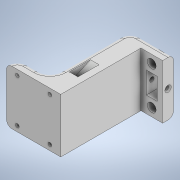
# Autodesk Inventor part: Joint_Tubes_1_2
Saved by Autodesk Inventor 2022.3 (Build 263350000, 350)
## iProperties
Created: 2023-03-29
Part Number: Joint_Tubes_1_2
Material: Generic
Document SubType Name: Modeling
Designer: Manuel Hueso Béjar
Density: 1 g/cm^3
Appearance: Default
Author: Manuel Hueso Béjar
Autodesk Inventor part; units mm, degrees
ref_plane "YZ Plane" through (0, 0, 0) normal (1, 0, 0) x (0, 1, 0)
ref_plane "XZ Plane" through (0, 0, 0) normal (0, 1, 0) x (-1, 0, 0)
ref_plane "XY Plane" through (0, 0, 0) normal (0, 0, 1) x (1, 0, 0)
sketch "Sketch1" plane through (0, 0, 0) normal (0, 1, 0) x (-1, 0, 0)
  line L0 (-10, 37) -> (10, 37)
  line L1 (10, 37) -> (10, -37)
  line L2 (10, -37) -> (-10, -37)
  line L3 (-10, -37) -> (-10, 37)
  line L4 (-10, 37) -> (10, -37) construction
  line L5 (10, 37) -> (-10, -37) construction
  line L6 (-10, 37) -> (40, 37)
  line L7 (40, 37) -> (40, 27)
  line L8 (40, 27) -> (-10, 27)
  line L9 (-10, 27) -> (-10, 37)
  line L10 (10, -37) -> (-30, -37)
  line L11 (-30, -37) -> (-30, -47)
  line L12 (-30, -47) -> (10, -47)
  line L13 (10, -47) -> (10, -37)
  point P0 (0, 0)
  point P1 (-10, -37)
  point P2 (10, 27)
  dimension "d0" = 20
  dimension "d1" = 74
  dimension "d2" = 50
  dimension "d3" = 10
  dimension "d4" = 40
  dimension "d5" = 10
  constraints: 28 end point, 6 parallel, 3 horizontal, 3 perpendicular, 2 midpoint
  measures "d0" distance of L1.end L2.end
  measures "d1" distance of L0.end L1.end
  measures "d2" distance of L7.end L8.end
  measures "d3" distance of L6.end L7.end
  measures "d4" distance of L12.end L11.end
  measures "d5" distance of L11.end L10.end
extrude "Extrusion1" add sketch "Sketch1" along normal blind 50
fillet "Fillet1" radius 10 2 edges at (-10, 25, -47) (-10, 25, 27)
fillet "Fillet2" radius 5 12 edges at (15, 50, -47) (-10, 50, -9.9999) (-12.9289, 50, 24.0711) (-29.9999, 50, 27) (-7.0711, 50, -44.0711) (-7.0711, 0, -44.0711) (-10, 0, -9.9999) (-12.9289, 0, 24.0711) (-29.9999, 0, 27) (15, 0, -47) (-40, 50, 32) (-40, 0, 32)
fillet "Fillet3" radius 10 3 edges at (-38.5355, 48.5355, 28.4645) (-38.5355, 1.4645, 28.4645) (-40, 25, 27)
sketch "Sketch2" plane through (10, 0, 37) normal (0, 0, 1) x (1, 0, 0)
  line L0 (0, 50) -> (-10, 50)
  line L1 (-10, 50) -> (-10, 45)
  line L2 (-10, 45) -> (0, 45)
  line L3 (0, 45) -> (0, 50)
  line L4 (-10, 0) -> (-10, 5) projected
  line L5 (0, 0) -> (-10, 0)
  line L6 (-10, 0) -> (-10, 5)
  line L7 (-10, 5) -> (0, 5)
  line L8 (0, 5) -> (0, 0)
  line L9 (0, 50) -> (-40, 50)
  line L10 (-40, 50) -> (-40, 45)
  line L11 (-40, 45) -> (0, 45)
  line L12 (0, 45) -> (0, 50)
  line L13 (0, 0) -> (-40, 0)
  line L14 (-40, 0) -> (-40, 5)
  line L15 (-40, 5) -> (0, 5)
  line L16 (0, 5) -> (0, 0)
  circle A0 centre (-10, 5) radius 1.7
  circle A1 centre (-10, 45) radius 1.7
  circle A2 centre (-40, 5) radius 1.7
  circle A3 centre (-40, 45) radius 1.7
  dimension "d11" = 10
  dimension "d12" = 5
  dimension "d13" = 10
  dimension "d14" = 5
  dimension "d15" = 40
  dimension "d16" = 5
  dimension "d17" = 40
  dimension "d18" = 5
  dimension "d19" = 3.4
  dimension "d20" = 3.4
  dimension "d21" = 3.4
  dimension "d22" = 3.4
  constraints: 32 end point, 8 parallel, 4 centre point, 4 coincident, 4 horizontal, 4 perpendicular
  measures "d11" distance of L2.end L1.end
  measures "d12" distance of L1.end L0.end
  measures "d13" distance of L4.end L7.end
  measures "d14" distance of L5.end L4.end
  measures "d15" distance of L11.end L10.end
  measures "d16" distance of L10.end L9.end
  measures "d17" distance of L14.end L15.end
  measures "d18" distance of L13.end L14.end
  measures "d19" diameter of A0
  measures "d20" diameter of A1
  measures "d21" diameter of A2
  measures "d22" diameter of A3
extrude "Extrusion2" cut sketch "Sketch2" against normal up to surface (10 mm away) contours A1 L2 L1 | L1 L11 A1 | A1 L11 L2 | A3 L11 L10 | L10 L11 A3 | A0 L15 L4 | L4 L7 A0 | L15 A0 L7 | A2 L15 L14 | L14 L15 A2
sketch "Sketch3" plane through (-20, 5, 27) normal (0, 0, -1) x (-1, 0, 0)
  circle A0 centre (10, 40) radius 1.7 projected
  arc A1 (10, 1.7) -> (8.3, 0) centre (10, 0) ccw projected
  line L0 (10, 40) -> (10, 0)
  point P0 (-20, -5)
  constraints: 2 end point, 1 vertical
hole "Hole1" at (-30, 45, 27) at (-30, 5, 27) direction (0, 0, 1) diameter 3.4 depth 2.2 countersink diameter 6 countersink angle 90
sketch "Sketch4" plane through (0, 45, 27) normal (0, 0, 1) x (1, 0, 0)
  line L0 (-4, -4) -> (4, -4)
  line L1 (4, -4) -> (4, 4)
  line L2 (4, 4) -> (-4, 4)
  line L3 (-4, 4) -> (-4, -4)
  line L4 (30, 0) -> (0, 0) projected
  line L5 (-4, -4) -> (4, 4) construction
  line L6 (4, -4) -> (-4, 4) construction
  point P0 (0, -45)
  dimension "d32" = 8
  dimension "d33" = 8
  constraints: 12 end point, 2 midpoint, 2 parallel, 1 horizontal, 1 perpendicular
  measures "d32" distance of L2.end L1.end
  measures "d33" distance of L1.end L0.end
sketch "Sketch5" plane through (10, 0, 37) normal (1, 0, 0) x (0, 0, -1)
  line L0 (0, 45) -> (20, 45)
  line L1 (20, 45) -> (20, 50)
  line L2 (20, 50) -> (0, 50)
  line L3 (0, 50) -> (0, 45)
  line L4 (20, 47.5) -> (40, 47.5)
  line L5 (40, 47.5) -> (40, 56.5)
  line L6 (40, 56.5) -> (20, 56.5)
  line L7 (20, 56.5) -> (20, 47.5)
  line L8 (20, 47.5) -> (40, 56.5)
  line L9 (0, 50) -> (74, 50) projected
  line L10 (0, 0) -> (0, 50) projected
  line L11 (20, 47.5) -> (10, 47.5)
  point P0 (37, 0)
  dimension "d34" = 20
  dimension "d35" = 5
  dimension "d36" = 20
  dimension "d37" = 9
  dimension "d38" = 0
  dimension "d39" = 0
  constraints: 20 end point, 4 parallel, 3 horizontal, 2 perpendicular, 1 midpoint, 1 other
  measures "d34" distance of L2.end L1.end
  measures "d35" distance of L1.end L0.end
  measures "d36" distance of L6.end L5.end
  measures "d37" distance of L5.end L4.end
  measures "d38" vertical extent of L2
  measures "d39" distance between parallel lines of L10 L3
sweep "Sweep1" cut profiles "Sketch4" path "Sketch5" path curves L11 L8
sketch "Sketch6" plane through (0, 5, 27) normal (0, 0, 1) x (1, 0, 0)
  line L0 (-4, -4) -> (4, -4)
  line L1 (4, -4) -> (4, 4)
  line L2 (4, 4) -> (-4, 4)
  line L3 (-4, 4) -> (-4, -4)
  line L4 (-10, 0) -> (0, 0) projected
  line L5 (-4, -4) -> (4, 4) construction
  line L6 (4, -4) -> (-4, 4) construction
  point P0 (0, -5)
  dimension "d42" = 8
  dimension "d43" = 8
  constraints: 12 end point, 2 midpoint, 2 parallel, 1 horizontal, 1 perpendicular
  measures "d42" distance of L2.end L1.end
  measures "d43" distance of L1.end L0.end
sketch "Sketch7" plane through (10, 0, 37) normal (1, 0, 0) x (0, 0, -1)
  line L0 (5, 0) -> (0, 0) projected
  line L1 (0, 0) -> (20, 0)
  line L2 (20, 0) -> (20, 5)
  line L3 (20, 5) -> (0, 5)
  line L4 (0, 5) -> (0, 0)
  line L5 (20, 2.5) -> (10, 2.5)
  line L6 (20, 2.5) -> (40, 2.5)
  line L7 (40, 2.5) -> (40, -6.5)
  line L8 (40, -6.5) -> (20, -6.5)
  line L9 (20, -6.5) -> (20, 2.5)
  line L10 (20, 2.5) -> (40, -6.5)
  point P0 (37, 0)
  dimension "d44" = 20
  dimension "d45" = 5
  dimension "d46" = 20
  dimension "d47" = 9
  constraints: 20 end point, 4 parallel, 3 horizontal, 2 perpendicular, 1 midpoint
  measures "d44" distance of L3.end L2.end
  measures "d45" distance of L2.end L1.end
  measures "d46" distance of L7.end L8.end
  measures "d47" distance of L6.end L7.end
sweep "Sweep2" cut profiles "Sketch6" path "Sketch7" path curves L5 L10
sketch "Sketch8" plane through (10, 0, -37) normal (0, 0, 1) x (1, 0, 0)
  line L0 (0, 50) -> (20, 50) projected
  line L1 (0, 0) -> (0, 50) projected
  line L2 (20, 50) -> (0, 50)
  line L3 (0, 50) -> (0, 0)
  line L4 (0, 0) -> (20, 0)
  line L5 (20, 0) -> (20, 50)
  line L6 (10, 50) -> (10, 0)
  line L7 (15, 15) -> (5, 15)
  line L8 (5, 15) -> (5, 35)
  line L9 (5, 35) -> (15, 35)
  line L10 (15, 35) -> (15, 15)
  line L11 (15, 15) -> (5, 35) construction
  line L12 (5, 15) -> (15, 35) construction
  line L13 (10, 50) -> (10, 35)
  line L14 (10, 0) -> (10, 15)
  circle A0 centre (10, 42.5) radius 4
  circle A1 centre (10, 7.5) radius 4
  point P0 (-10, 0)
  point P1 (10, 25)
  dimension "d50" = 10
  dimension "d51" = 20
  dimension "d52" = 8
  dimension "d53" = 8
  constraints: 26 end point, 9 midpoint, 4 parallel, 2 centre point, 2 horizontal, 2 perpendicular
  measures "d50" distance of L8.end L9.end
  measures "d51" distance of L7.end L8.end
  measures "d52" diameter of A0
  measures "d53" diameter of A1
extrude "Extrusion3" cut sketch "Sketch8" against normal through all contours A0 L6 | L6 A0 | A1 L6 | L6 A1
extrude "Extrusion4" cut sketch "Sketch8" against normal through all contours L9 L10 L7 L6 | L6 L7 L8 L9
sketch "Sketch9" plane through (0, 5, -47) normal (0, 0, -1) x (-1, 0, 0)
  circle A0 centre (-20, 2.5) radius 4 projected
  circle A1 centre (-20, 2.5) radius 6
  arc A2 (-23.1225, 40) -> (-16.8775, 40) centre (-20, 37.5) ccw projected
  circle A3 centre (-20, 37.5) radius 6
  point P0 (0, -5)
  dimension "d58" = 12
  dimension "d59" = 12
  constraints: 2 centre point, 2 coincident
  measures "d58" diameter of A1
  measures "d59" diameter of A3
extrude "Extrusion5" cut sketch "Sketch9" against normal blind 2 contours A0 | A1 | A3
sketch "Sketch10" plane through (30, 0, -37) normal (1, 0, 0) x (0, 0, -1)
  line L0 (10, 15) -> (10, 35) projected
  line L1 (0, 15) -> (10, 15) projected
  line L2 (0, 35) -> (0, 15) projected
  line L3 (0, 35) -> (10, 35) projected
  line L4 (0, 35) -> (10, 15)
  line L5 (5, 25) -> (10, 25)
  point P0 (-37, 0)
  constraints: 4 end point, 2 midpoint
hole "Hole2" at (30, 25, -42) direction (-1, 0, 0) diameter 3.4 depth 5 countersink diameter 5.9 countersink angle 90
sketch "Sketch11" plane through (15, 15, -37) normal (1, 0, 0) x (0, 0, -1)
  circle A0 centre (5, 10) radius 1.7 projected
  line L0 (5, 10) -> (5, 11.7)
  point P0 (-37, -15)
  constraints: 2 end point, 1 vertical, 1 vertical alignment, 1 other
hole "Hole3" at (15, 25, -42) direction (-1, 0, 0) diameter 3.4 depth 12 counterbore diameter 4.1 counterbore depth 5.1
body "Solid1"
